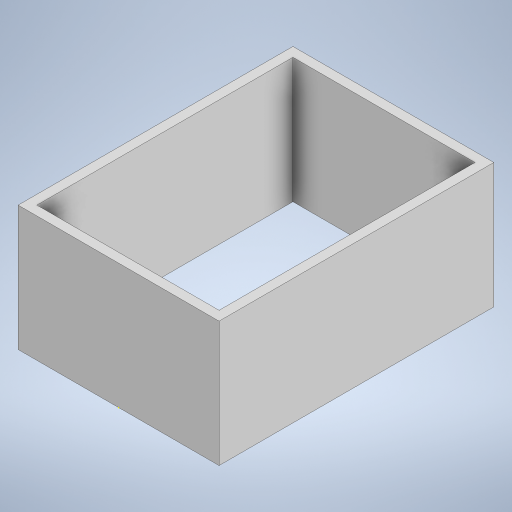
# Autodesk Inventor part: Case
Saved by Autodesk Inventor 2023 (Build 270158000, 158)
## iProperties
Created: 2022-04-12
Part Number: Case
Material: Generic
Document SubType Name: Modeling
Designer: cooki
Density: 1 g/cm^3
Appearance: Default
Author: cooki
Autodesk Inventor part; units mm, degrees
ref_plane "YZ Plane" through (0, 0, 0) normal (1, 0, 0) x (0, 1, 0)
ref_plane "XZ Plane" through (0, 0, 0) normal (0, 1, 0) x (-1, 0, 0)
ref_plane "XY Plane" through (0, 0, 0) normal (0, 0, 1) x (1, 0, 0)
sketch "Sketch1" plane through (0, 0, 0) normal (0, 1, 0) x (-1, 0, 0)
  line L0 (37, 52) -> (-37, 52)
  line L1 (-37, 52) -> (-37, -52)
  line L2 (-37, -52) -> (37, -52)
  line L3 (37, -52) -> (37, 52)
  line L4 (40.81, 55.81) -> (-40.81, 55.81)
  line L5 (-40.81, 55.81) -> (-40.81, -55.81)
  line L6 (-40.81, -55.81) -> (40.81, -55.81)
  line L7 (40.81, -55.81) -> (40.81, 55.81)
  point P0 (0, 0)
  point P1 (0, -52)
  point P2 (37, 0)
  dimension "d0" = 74
  dimension "d1" = 104
  dimension "d2" = 3.81
  constraints: 16 end point, 4 parallel, 2 midpoint, 2 perpendicular, 1 horizontal, 1 horizontal alignment, 1 vertical alignment, 3 other
  measures "d0" distance between parallel lines of L1 L3
  measures "d1" distance between parallel lines of L0 L2
  measures "d2" distance between parallel lines of L3 L7
extrude "Extrusion1" add sketch "Sketch1" along normal blind 50.8
sketch "Sketch2" plane through (-40.81, 0, 55.81) normal (0, 0, 1) x (1, 0, 0)
  point P0 (40.81, 0)
body "Solid1"
